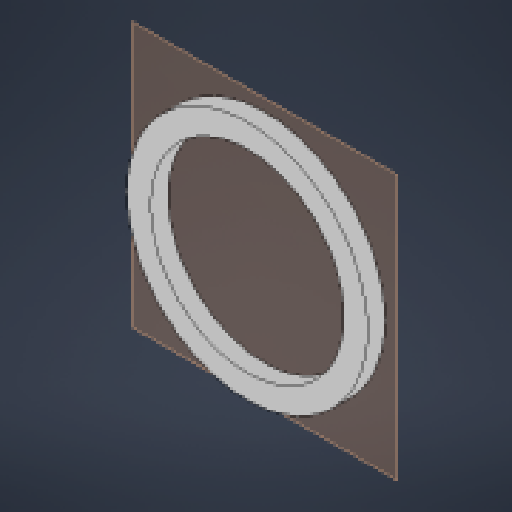
# Autodesk Inventor part: TopSpacer
Saved by Autodesk Inventor 2024 (Build 280153000, 153)
## iProperties
Created: 2023-10-21
Part Number: TopSpacer
Material: Generic
Document SubType Name: Modeling
Designer: range
Density: 1 g/cm^3
Appearance: Default
Author: range
Autodesk Inventor part; units mm, degrees
ref_plane "YZ Plane" through (0, 0, 0) normal (1, 0, 0) x (0, 1, 0)
ref_plane "XZ Plane" through (0, 0, 0) normal (0, 1, 0) x (-1, 0, 0)
ref_plane "XY Plane" through (0, 0, 0) normal (0, 0, 1) x (1, 0, 0)
ref_plane "Work Plane1" through (0, 0, 0) normal (0, 0, 1) x (1, 0, 0)
sketch "Sketch1" plane through (0, 0, 0) normal (0, 0, 1) x (1, 0, 0)
  circle A0 centre (0, -55.5) radius 5.1943 projected
  circle A1 centre (-55.5, 0) radius 5.1943 projected
  circle A2 centre (0, 55.5) radius 5.1943 projected
  circle A3 centre (55.5, 0) radius 5.1943 projected
  circle A4 centre (0, 0) radius 61.5 projected
  circle A5 centre (0, 0) radius 49.5 projected
  line L0 (-2.0207, 52) -> (-4.0415, 55.5)
  line L1 (-4.0415, 55.5) -> (-2.0207, 59)
  line L2 (-2.0207, 59) -> (2.0207, 59)
  line L3 (2.0207, 59) -> (4.0415, 55.5)
  line L4 (4.0415, 55.5) -> (2.0207, 52)
  line L5 (2.0207, 52) -> (-2.0207, 52)
  line L6 (0, 55.5) -> (0, 52) construction
  line L7 (-52, -2.0207) -> (-55.5, -4.0415)
  line L8 (-55.5, -4.0415) -> (-59, -2.0207)
  line L9 (-59, -2.0207) -> (-59, 2.0207)
  line L10 (-59, 2.0207) -> (-55.5, 4.0415)
  line L11 (-55.5, 4.0415) -> (-52, 2.0207)
  line L12 (-52, 2.0207) -> (-52, -2.0207)
  line L13 (2.0207, -52) -> (4.0415, -55.5)
  line L14 (4.0415, -55.5) -> (2.0207, -59)
  line L15 (2.0207, -59) -> (-2.0207, -59)
  line L16 (-2.0207, -59) -> (-4.0415, -55.5)
  line L17 (-4.0415, -55.5) -> (-2.0207, -52)
  line L18 (-2.0207, -52) -> (2.0207, -52)
  line L19 (52, 2.0207) -> (55.5, 4.0415)
  line L20 (55.5, 4.0415) -> (59, 2.0207)
  line L21 (59, 2.0207) -> (59, -2.0207)
  line L22 (59, -2.0207) -> (55.5, -4.0415)
  line L23 (55.5, -4.0415) -> (52, -2.0207)
  line L24 (52, -2.0207) -> (52, 2.0207)
  circle A6 centre (0, 55.5) radius 5.1943
  circle A7 centre (-39.2444, 39.2444) radius 5.1943
  line L25 (-39.2444, 39.2444) -> (0, 0)
  line L26 (0, 55.5) -> (0, -55.5)
  circle A8 centre (-39.2444, -39.2444) radius 5.1943
  circle A9 centre (39.2444, -39.2444) radius 5.1943
  circle A10 centre (39.2444, 39.2444) radius 5.1943
  point P0 (-52, 0)
  point P1 (0, -52)
  point P2 (52, 0)
  dimension "d2" = 7
  dimension "d5" = 360
  dimension "d11" = 45
  dimension "d12" = 10.3886
  dimension "d13" = 55.5
  dimension "d16" = 360
  constraints: 54 end point, 5 centre point, 2 coincident, 2 vertical, 1 concentric, 1 midpoint, 75 other
  measures "d2" distance between parallel lines of L4 L1
  measures "d11" angle of L25 L26
  measures "d12" diameter of A7
  measures "d13" distance of L25.start L25.end
extrude "Extrusion1" add sketch "Sketch1" along normal blind 8.89 contours A0 | A1 | A2 | A3 | A4 | L0 L1 L2 L3 L4 L5 | L7 L8 L9 L10 L11 L12 | L13 L14 L15 L16 L17 L18 | L19 L20 L21 L22 L23 L24 | A7 | A8 | A9 | A10
extrude "Extrusion2" cut sketch "Sketch1" along normal blind 6.35 contours L0 L1 L2 L3 L4 L5 | L7 L8 L9 L10 L11 L12 | L13 L14 L15 L16 L17 L18 | L19 L20 L21 L22 L23 L24
body "Solid1"
